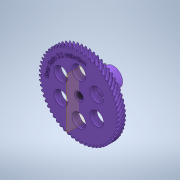
# Autodesk Inventor part: Spur Gear1
Saved by Autodesk Inventor 2020.2 (Build 242310000, 310)
## iProperties
CustomPartVersion: 1
Created: 2019-11-22
Part Number: Spur Gear1
Material: Steel
Document SubType Name: Modeling
Designer: steele
Categories: <?xml version="1.0" encoding="UTF-16"?> <MemberInstance><Categories><FamilyTemplate><FamilyTemplateParameter ValueType="xs:double" Id="1" ObjectReferenceKey="da_z" ObjectType="kUserParameterObject"/><FamilyTemplateParameter ValueType="xs:double" Id="2" ObjectReferenceKey="da_b" ObjectType="kUserParameterObject"/><FamilyTemplateParameter ValueType="xs:double" Id="3" ObjectReferenceKey="da_beta" ObjectType="kUserParameterObject"/><FamilyTemplateParameter ValueType="xs:double" Id="4" ObjectReferenceKey="da_da" ObjectType="kUserParameterObject"/><FamilyTemplateParameter ValueType="xs:double" Id="5" ObjectReferenceKey="da_aw" ObjectType="kUserParameterObject"/><FamilyTemplateParameter ValueType="xs:string" Id="6" ObjectReferenceKey="EAIAABAAAAC/AAAAAAAAAIAAAAAAAAAA" ObjectType="83910656" SubObjectId="SurfaceGeometry"/></FamilyTemplate><ParamToTemplateMap><ParamToTemplate CategoryParameter="//CategoryParameter[@InternalName='046C89C9-8512-4d59-83FE-43B91F4F132A']" TemplateParameter="1"/><ParamToTemplate CategoryParameter="//CategoryParameter[@InternalName='2552DF32-E462-4b46-AEBF-C6C7768E72AC']" TemplateParameter="2"/><ParamToTemplate CategoryParameter="//CategoryParameter[@InternalName='C9EE641D-15FC-4fae-A226-E94C4372FDD7']" TemplateParameter="3"/><ParamToTemplate><ParamToTemplate CategoryParameter="//CategoryParameter[@InternalName='00B6519A-459B-49c7-AD84-2E56D39A5744']" ConstantValue="0.000000"/></ParamToTemplate><ParamToTemplate><ParamToTemplate CategoryParameter="//CategoryParameter[@InternalName='04B31F0E-C7A6-4894-AA32-9629BEFACF47']" ConstantValue="1.000000"/></ParamToTemplate><ParamToTemplate><ParamToTemplate CategoryParameter="//CategoryParameter[@InternalName='43CBEC2E-7847-49e7-A936-2F7889FCB2D9']" ConstantValue="0.250000"/></ParamToTemplate><ParamToTemplate><ParamToTemplate CategoryParameter="//CategoryParameter[@InternalName='B1EFC894-105D-4ebd-86BF-FA20ED196853']" ConstantValue="0.350000"/></ParamToTemplate><ParamToTemplate><ParamToTemplate CategoryParameter="//CategoryParameter[@InternalName='51175063-3D10-4879-93E8-6246FE8B403D']" ConstantValue="2061532430.657340"/></ParamToTemplate><ParamToTemplate><ParamToTemplate CategoryParameter="//CategoryParameter[@InternalName='A3A52E27-4454-46a9-B0BD-C932399B70AF']" ConstantValue="0.300000"/></ParamToTemplate><ParamToTemplate><ParamToTemplate CategoryParameter="//CategoryParameter[@InternalName='91B76062-C214-41d9-B1B9-14D2AB99603D']" ConstantValue="0.127000"/></ParamToTemplate><ParamToTemplate><ParamToTemplate CategoryParameter="//CategoryParameter[@InternalName='374E806E-8B8A-4dda-A9AA-1039D6500AD2']" ConstantValue="7.874016"/></ParamToTemplate><ParamToTemplate><ParamToTemplate CategoryParameter="//CategoryParameter[@InternalName='2D373A89-B862-43d6-8D0B-0CBF12AB9F6C']" ConstantValue="0.349066"/></ParamToTemplate><ParamToTemplate CategoryParameter="//CategoryParameter[@InternalName='37777632-D6A2-4fac-9D53-DB8ACD95C989']" TemplateParameter="4"/><ParamToTemplate CategoryParameter="//CategoryParameter[@InternalName='FD1017F1-B727-4f7e-9707-0F86F1FF9423']" TemplateParameter="5"/><ParamToTemplate><ParamToTemplate CategoryParameter="//CategoryParameter[@InternalName='9E1B4470-B2D3-4ff1-B813-535BB4CDF51A']" ConstantValue="3523220.976809"/></ParamToTemplate><ParamToTemplate><ParamToTemplate CategoryParameter="//CategoryParameter[@InternalName='F8452263-BFF6-458c-9FB1-07C4B99E95CD']" ConstantValue="11397033.805607"/></ParamToTemplate><ParamToTemplate><ParamToTemplate CategoryParameter="//CategoryParameter[@InternalName='3E3BB259-FD49-497f-8171-6EBC954A3479']" ConstantValue="2.000000"/></ParamToTemplate><ParamToTemplate CategoryParameter="//CategoryParameter[@InternalName='27C3BAF2-7550-4e4b-AE2C-0DB134B7D9B7']" TemplateParameter="6"/></ParamToTemplateMap><Category DisplayName="Gear" InternalName="DC85795E-93AB-48d5-8EEE-5A27447B64BD" Mnemonic="Gear"><CategoryParameter DisplayName="z" InternalName="046C89C9-8512-4d59-83FE-43B91F4F132A" Mnemonic="z"/><CategoryParameter DisplayName="b" InternalName="2552DF32-E462-4b46-AEBF-C6C7768E72AC" Mnemonic="b"/><CategoryParameter DisplayName="||b|" InternalName="C9EE641D-15FC-4fae-A226-E94C4372FDD7" Mnemonic="beta"/><CategoryParameter DisplayName="x" InternalName="00B6519A-459B-49c7-AD84-2E56D39A5744" Mnemonic="x"/><CategoryParameter DisplayName="a*" InternalName="04B31F0E-C7A6-4894-AA32-9629BEFACF47" Mnemonic="a"/><CategoryParameter DisplayName="c*" InternalName="43CBEC2E-7847-49e7-A936-2F7889FCB2D9" Mnemonic="c"/><CategoryParameter DisplayName="r|.f|*" InternalName="B1EFC894-105D-4ebd-86BF-FA20ED196853" Mnemonic="rf"/><CategoryParameter DisplayName="E" InternalName="51175063-3D10-4879-93E8-6246FE8B403D" Mnemonic="E"/><CategoryParameter DisplayName="||m|" InternalName="A3A52E27-4454-46a9-B0BD-C932399B70AF" Mnemonic="mi"/><Category DisplayName="SpurGear" InternalName="26C5A22E-A91E-4dfd-A3B3-23CCAFAE1764" Mnemonic="SpurGear"><CategoryParameter DisplayName="m" InternalName="91B76062-C214-41d9-B1B9-14D2AB99603D" Mnemonic="m"/><CategoryParameter DisplayName="P" InternalName="374E806E-8B8A-4dda-A9AA-1039D6500AD2" Mnemonic="PP"/><CategoryParameter DisplayName="||a|" InternalName="2D373A89-B862-43d6-8D0B-0CBF12AB9F6C" Mnemonic="alpha"/><CategoryParameter DisplayName="d|.a|" InternalName="37777632-D6A2-4fac-9D53-DB8ACD95C989" Mnemonic="da"/><CategoryParameter DisplayName="a|.w|" InternalName="FD1017F1-B727-4f7e-9707-0F86F1FF9423" Mnemonic="aw"/><CategoryParameter DisplayName="||s||.Flim|" InternalName="9E1B4470-B2D3-4ff1-B813-535BB4CDF51A" Mnemonic="sFlim"/><CategoryParameter DisplayName="||s||.Hlim|" InternalName="F8452263-BFF6-458c-9FB1-07C4B99E95CD" Mnemonic="sHlim"/><CategoryParameter DisplayName="type" InternalName="3E3BB259-FD49-497f-8171-6EBC954A3479" Mnemonic="type"/><CategoryParameter DisplayName="PitchDiameter" InternalName="27C3BAF2-7550-4e4b-AE2C-0DB134B7D9B7" Mnemonic="IDS_PITCHDIAM"/></Category></Category></Categories></MemberInstance>
Density: 1 g/cm^3
Appearance: Violet
Author: steele
Autodesk Inventor part; units mm, degrees
(part 1 of 2)
ref_plane "XZ Plane" through (0, 0, 0) normal (0, 1, 0) x (-1, 0, 0)
ref_plane "XY Plane" through (0, 0, 0) normal (0, 0, 1) x (1, 0, 0)
sketch "Sketch1" plane through (0, 0, 0) normal (0, 0, 1) x (1, 0, 0)
  circle A0 centre (0, 0) radius 55.1515
  dimension "d0" = 110.3031
  constraints: 1 centre point
  measures "d0" diameter of A0
extrude "Extrusion1" add sketch "Sketch1" along normal blind 9.525
sketch "Sketch2" plane through (0, 0, 0) normal (0, 0, -1) x (-1, 0, 0)
  circle A0 centre (0, 0) radius 55.1515 projected
  circle A1 centre (0, 0) radius 53.8815
  dimension "d3" = 107.7631
  constraints: 1 centre point, 1 coincident
  measures "d3" diameter of A1
surface extrude "Pitch Diameter" sketch "Sketch2" against normal through all shown no curves A1
ref_plane "Work Plane1" through (0, 0, 0) normal (1, 0, 0) x (0, 1, 0)
ref_plane "Work Plane2" through (0, 0, 0) normal (0.9986295, 0.052336, 0) x (0, 0, 1)
ref_plane "Work Plane3" through (0, 0, 4.7625) normal (0, 0, -1) x (-1, 0, 0)
spur gear teeth "Spur Gear" teeth 60 pitch diameter 107.7631 tip diameter 110.3031 root diameter 104.5881 face width 9.525 helix angle 45 hand left start plane through (0, 0, 0) normal (0, 0, -1) x (-1, 0, 0)
sketch "Sketch3" plane through (0, 0, 0) normal (0, 0, -1) x (-1, 0, 0)
  circle A0 centre (0, 0) radius 12.7
  dimension "d20" = 25.4
  constraints: 1 centre point, 1 coincident
  measures "d20" diameter of A0
extrude "Extrusion2" add sketch "Sketch3" along normal blind 38.1
sketch "Sketch4" plane through (0, 0, -38.1) normal (0, 0, -1) x (-1, 0, 0)
  circle A0 centre (0, 0) radius 4.7625
  dimension "d23" = 9.525
  constraints: 1 centre point, 1 coincident
  measures "d23" diameter of A0
extrude "Extrusion3" cut sketch "Sketch4" against normal through all
sketch "Sketch5" plane through (0, 0, 0) normal (0, 0, -1) x (-1, 0, 0)
  circle A0 centre (0, 0) radius 4.7625 projected
  circle A1 centre (0, 28.575) radius 9.525
  circle A2 centre (-24.7467, 14.2875) radius 9.525
  circle A3 centre (-24.7467, -14.2875) radius 9.525
  circle A4 centre (0, -28.575) radius 9.525
  circle A5 centre (24.7467, -14.2875) radius 9.525
  circle A6 centre (24.7467, 14.2875) radius 9.525
  dimension "d27" = 19.05
  dimension "d30" = 360
  constraints: 6 centre point, 2 coincident, 17 other
  measures "d27" diameter of A1
extrude "Extrusion4" cut sketch "Sketch5" against normal through all contours A1 | A2 | A3 | A4 | A5 | A6
fillet "Fillet1" radius 1.5875 2 edges at (4.7625, 0, 9.525) (4.7625, 0, -38.1)
sketch "Sketch6" plane through (0, 0, 9.525) normal (0, 0, 1) x (1, 0, 0)
  circle A0 centre (0, 0) radius 4.7625 construction
  circle A1 centre (0, 0) radius 44.45 construction
  spline S0 degree 2 poles (-41.7293, 2.6333) (-41.7593, 2.0949) (-42.1378, 1.2212) (-42.4885, 0.9192) knots 0 0 0 1 2 2 2
  spline S1 degree 2 poles (-42.4885, 0.9192) (-42.8434, 0.6173) (-43.8571, 0.3315) (-44.5024, 0.3674) knots 0 0 0 1 2 2 2
  spline S2 degree 2 poles (-44.5024, 0.3674) (-45.1149, 0.4015) (-46.0657, 0.8007) (-46.3931, 1.1406) knots 0 0 0 1 2 2 2
  spline S3 degree 2 poles (-46.3931, 1.1406) (-46.7089, 1.4674) (-47.0203, 2.3918) (-46.9903, 2.9302) knots 0 0 0 1 2 2 2
  spline S4 degree 2 poles (-46.9903, 2.9302) (-46.9759, 3.1892) (-46.8759, 3.6536) (-46.7982, 3.8637) knots 0 0 0 1 2 2 2
  spline S5 degree 2 poles (-46.7982, 3.8637) (-46.7393, 4.0336) (-46.5351, 4.4428) (-46.4622, 4.5666) knots 0 0 0 1 2 2 2
  line L0 (-46.4622, 4.5666) -> (-45.6484, 4.5213)
  line L1 (-45.6484, 4.5213) -> (-45.6516, 4.4637)
  spline S6 degree 2 poles (-45.6516, 4.4637) (-45.7697, 4.3425) (-45.9859, 4.0865) (-46.1148, 3.8463) knots 0 0 0 1 2 2 2
  spline S7 degree 2 poles (-46.1148, 3.8463) (-46.229, 3.6465) (-46.3941, 3.1238) (-46.411, 2.8196) knots 0 0 0 1 2 2 2
  spline S8 degree 2 poles (-46.411, 2.8196) (-46.4517, 2.088) (-45.4005, 1.1224) (-44.4839, 1.0714) knots 0 0 0 1 2 2 2
  spline S9 degree 2 poles (-44.4839, 1.0714) (-43.9742, 1.0431) (-43.1964, 1.2389) (-42.9208, 1.4504) knots 0 0 0 1 2 2 2
  spline S10 degree 2 poles (-42.9208, 1.4504) (-42.6456, 1.6536) (-42.3359, 2.2548) (-42.3144, 2.6412) knots 0 0 0 1 2 2 2
  spline S11 degree 2 poles (-42.3144, 2.6412) (-42.2986, 2.9248) (-42.3492, 3.4966) (-42.4207, 3.6943) knots 0 0 0 1 2 2 2
  line L2 (-42.4207, 3.6943) -> (-43.7319, 3.7673)
  line L3 (-43.7319, 3.7673) -> (-43.7973, 2.5917)
  line L4 (-43.7973, 2.5917) -> (-44.3892, 2.6247)
  line L5 (-44.3892, 2.6247) -> (-44.2867, 4.4661)
  line L6 (-44.2867, 4.4661) -> (-42.0713, 4.3428)
  spline S12 degree 2 poles (-42.0713, 4.3428) (-42.0208, 4.2122) (-41.8683, 3.7667) (-41.8252, 3.5787) knots 0 0 0 1 2 2 2
  spline S13 degree 2 poles (-41.8252, 3.5787) (-41.7651, 3.3239) (-41.7136, 2.917) (-41.7293, 2.6333) knots 0 0 0 1 2 2 2
  spline S14 degree 2 poles (-41.2786, 6.7356) (-41.4197, 5.8327) (-42.5875, 4.9985) (-43.523, 5.1447) knots 0 0 0 1 2 2 2
  spline S15 degree 2 poles (-43.523, 5.1447) (-44.4422, 5.2883) (-45.3816, 6.4226) (-45.2602, 7.1995) knots 0 0 0 1 2 2 2
  spline S16 degree 2 poles (-45.2602, 7.1995) (-45.2056, 7.5493) (-44.9177, 8.0584) (-44.671, 8.224) knots 0 0 0 1 2 2 2
  spline S17 degree 2 poles (-44.671, 8.224) (-44.4236, 8.3937) (-43.7676, 8.5121) (-43.3162, 8.4415) knots 0 0 0 1 2 2 2
  line L7 (-43.3162, 8.4415) -> (-42.9704, 8.3875)
  line L8 (-42.9704, 8.3875) -> (-43.3778, 5.7803)
  spline S18 degree 2 poles (-43.3778, 5.7803) (-42.723, 5.678) (-41.9245, 6.2282) (-41.833, 6.8139) knots 0 0 0 1 2 2 2
  spline S19 degree 2 poles (-41.833, 6.8139) (-41.8006, 7.0214) (-41.8312, 7.4386) (-41.879, 7.6128) knots 0 0 0 1 2 2 2
  spline S20 degree 2 poles (-41.879, 7.6128) (-41.9337, 7.7963) (-42.0391, 8.0545) (-42.0922, 8.1419) knots 0 0 0 1 2 2 2
  line L9 (-42.0922, 8.1419) -> (-42.0864, 8.1785)
  line L10 (-42.0864, 8.1785) -> (-41.395, 8.0705)
  spline S21 degree 2 poles (-41.395, 8.0705) (-41.3674, 7.9537) (-41.2894, 7.5998) (-41.2731, 7.4639) knots 0 0 0 1 2 2 2
  spline S22 degree 2 poles (-41.2731, 7.4639) (-41.2488, 7.2726) (-41.243, 6.9634) (-41.2786, 6.7356) knots 0 0 0 1 2 2 2
  spline S23 degree 2 poles (-43.5511, 7.8449) (-43.8086, 7.8768) (-44.1993, 7.8295) (-44.3413, 7.7475) knots 0 0 0 1 2 2 2
  spline S24 degree 2 poles (-44.3413, 7.7475) (-44.5008, 7.66) (-44.7053, 7.3377) (-44.7453, 7.0815) knots 0 0 0 1 2 2 2
  spline S25 degree 2 poles (-44.7453, 7.0815) (-44.7847, 6.8293) (-44.6895, 6.452) (-44.566, 6.2827) knots 0 0 0 1 2 2 2
  spline S26 degree 2 poles (-44.566, 6.2827) (-44.4378, 6.1168) (-44.0986, 5.9138) (-43.8618, 5.856) knots 0 0 0 1 2 2 2
  line L11 (-43.8618, 5.856) -> (-43.5511, 7.8449)
  spline S27 degree 2 poles (-40.8932, 10.8969) (-40.8561, 10.8071) (-40.7195, 10.5019) (-40.6893, 10.3672) knots 0 0 0 1 2 2 2
  spline S28 degree 2 poles (-40.6893, 10.3672) (-40.6419, 10.1816) (-40.6261, 9.8511) (-40.6953, 9.5714) knots 0 0 0 1 2 2 2
  spline S29 degree 2 poles (-40.6953, 9.5714) (-40.7517, 9.3436) (-41.0254, 8.9745) (-41.2198, 8.8573) knots 0 0 0 1 2 2 2
  spline S30 degree 2 poles (-41.2198, 8.8573) (-41.4082, 8.747) (-41.9003, 8.6779) (-42.1481, 8.7392) knots 0 0 0 1 2 2 2
  spline S31 degree 2 poles (-42.1481, 8.7392) (-42.5317, 8.8341) (-42.9951, 9.2923) (-43.0639, 9.6825) knots 0 0 0 1 2 2 2
  spline S32 degree 2 poles (-43.0639, 9.6825) (-43.1307, 10.0298) (-43.0289, 10.9037) (-42.9353, 11.4022) knots 0 0 0 1 2 2 2
  line L12 (-42.9353, 11.4022) -> (-43.0552, 11.4318)
  spline S33 degree 2 poles (-43.0552, 11.4318) (-43.2709, 11.4852) (-43.5713, 11.4196) (-43.6769, 11.3185) knots 0 0 0 1 2 2 2
  spline S34 degree 2 poles (-43.6769, 11.3185) (-43.7825, 11.2174) (-43.9155, 10.8856) (-43.961, 10.7018) knots 0 0 0 1 2 2 2
  spline S35 degree 2 poles (-43.961, 10.7018) (-44.0144, 10.486) (-44.0309, 9.8709) (-43.9792, 9.5485) knots 0 0 0 1 2 2 2
  line L13 (-43.9792, 9.5485) -> (-43.9881, 9.5126)
  line L14 (-43.9881, 9.5126) -> (-44.6235, 9.6698)
  spline S36 degree 2 poles (-44.6235, 9.6698) (-44.6289, 9.8535) (-44.5896, 10.5265) (-44.5115, 10.8422) knots 0 0 0 1 2 2 2
  spline S37 degree 2 poles (-44.5115, 10.8422) (-44.4165, 11.2259) (-44.1671, 11.7197) (-43.9598, 11.8889) knots 0 0 0 1 2 2 2
  spline S38 degree 2 poles (-43.9598, 11.8889) (-43.7576, 12.0552) (-43.2246, 12.1353) (-42.8769, 12.0493) knots 0 0 0 1 2 2 2
  line L15 (-42.8769, 12.0493) -> (-40.3473, 11.4234)
  line L16 (-40.3473, 11.4234) -> (-40.5016, 10.8)
  line L17 (-40.5016, 10.8) -> (-40.8932, 10.8969)
  line L18 (-41.4127, 11.0254) -> (-42.4397, 11.2796)
  spline S39 degree 2 poles (-42.4397, 11.2796) (-42.4751, 11.0508) (-42.5743, 10.3587) (-42.5628, 10.131) knots 0 0 0 1 2 2 2
  spline S40 degree 2 poles (-42.5628, 10.131) (-42.5482, 9.8645) (-42.3126, 9.4627) (-42.0328, 9.3935) knots 0 0 0 1 2 2 2
  spline S41 degree 2 poles (-42.0328, 9.3935) (-41.7131, 9.3144) (-41.3004, 9.5939) (-41.2154, 9.9376) knots 0 0 0 1 2 2 2
  spline S42 degree 2 poles (-41.2154, 9.9376) (-41.1432, 10.2293) (-41.2763, 10.7712) (-41.4127, 11.0254) knots 0 0 0 1 2 2 2
  line L19 (-42.4182, 15.1761) -> (-42.4284, 15.1448)
  spline S43 degree 2 poles (-42.4284, 15.1448) (-42.471, 15.0808) (-42.5288, 14.9308) (-42.5634, 14.8252) knots 0 0 0 1 2 2 2
  spline S44 degree 2 poles (-42.5634, 14.8252) (-42.6441, 14.5787) (-42.5877, 14.0231) (-42.4482, 13.7349) knots 0 0 0 1 2 2 2
  line L20 (-42.4482, 13.7349) -> (-39.8777, 12.8934)
  line L21 (-39.8777, 12.8934) -> (-40.0775, 12.2831)
  line L22 (-40.0775, 12.2831) -> (-43.7004, 13.469)
  line L23 (-43.7004, 13.469) -> (-43.5006, 14.0794)
  line L24 (-43.5006, 14.0794) -> (-42.9607, 13.9026)
  spline S45 degree 2 poles (-42.9607, 13.9026) (-43.1492, 14.3325) (-43.2291, 14.9088) (-43.1522, 15.1435) knots 0 0 0 1 2 2 2
  spline S46 degree 2 poles (-43.1522, 15.1435) (-43.1215, 15.2374) (-43.0829, 15.3288) (-43.052, 15.3836) knots 0 0 0 1 2 2 2
  line L25 (-43.052, 15.3836) -> (-42.4182, 15.1761)
  line L26 (-36.7442, 20.2855) -> (-37.1257, 19.496)
  line L27 (-37.1257, 19.496) -> (-39.6442, 18.9298)
  line L28 (-39.6442, 18.9298) -> (-39.9809, 18.2329)
  line L29 (-39.9809, 18.2329) -> (-38.161, 17.3535)
  line L30 (-38.161, 17.3535) -> (-38.4547, 16.7456)
  line L31 (-38.4547, 16.7456) -> (-43.0287, 18.9558)
  line L32 (-43.0287, 18.9558) -> (-42.4592, 20.1345)
  spline S47 degree 2 poles (-42.4592, 20.1345) (-42.2693, 20.5274) (-41.9279, 21.0163) (-41.6558, 21.182) knots 0 0 0 1 2 2 2
  spline S48 degree 2 poles (-41.6558, 21.182) (-41.3837, 21.3477) (-40.7638, 21.391) (-40.4043, 21.2173) knots 0 0 0 1 2 2 2
  spline S49 degree 2 poles (-40.4043, 21.2173) (-39.9039, 20.9755) (-39.4727, 20.1362) (-39.521, 19.62) knots 0 0 0 1 2 2 2
  line L33 (-39.521, 19.62) -> (-36.7442, 20.2855)
  spline S50 degree 2 poles (-40.6624, 20.5602) (-40.8625, 20.6569) (-41.2382, 20.6647) (-41.41, 20.5648) knots 0 0 0 1 2 2 2
  spline S51 degree 2 poles (-41.41, 20.5648) (-41.5579, 20.4763) (-41.7949, 20.1656) (-41.9167, 19.9135) knots 0 0 0 1 2 2 2
  line L34 (-41.9167, 19.9135) -> (-42.2086, 19.3093)
  line L35 (-42.2086, 19.3093) -> (-40.4888, 18.4783)
  line L36 (-40.4888, 18.4783) -> (-40.2308, 19.012)
  spline S52 degree 2 poles (-40.2308, 19.012) (-40.1037, 19.2752) (-39.994, 19.7388) (-40.0687, 19.9533) knots 0 0 0 1 2 2 2
  spline S53 degree 2 poles (-40.0687, 19.9533) (-40.1302, 20.1476) (-40.4252, 20.4456) (-40.6624, 20.5602) knots 0 0 0 1 2 2 2
  spline S54 degree 2 poles (-35.78, 22.6006) (-35.7713, 22.5039) (-35.7321, 22.1718) (-35.7434, 22.0342) knots 0 0 0 1 2 2 2
  spline S55 degree 2 poles (-35.7434, 22.0342) (-35.7535, 21.8429) (-35.837, 21.5228) (-35.9866, 21.2765) knots 0 0 0 1 2 2 2
  spline S56 degree 2 poles (-35.9866, 21.2765) (-36.1083, 21.0759) (-36.4796, 20.8053) (-36.7002, 20.7513) knots 0 0 0 1 2 2 2
  spline S57 degree 2 poles (-36.7002, 20.7513) (-36.913, 20.7023) (-37.4032, 20.7832) (-37.6214, 20.9156) knots 0 0 0 1 2 2 2
  spline S58 degree 2 poles (-37.6214, 20.9156) (-37.9593, 21.1206) (-38.2649, 21.6962) (-38.2141, 22.0892) knots 0 0 0 1 2 2 2
  spline S59 degree 2 poles (-38.2141, 22.0892) (-38.1742, 22.4406) (-37.8164, 23.2443) (-37.5783, 23.6921) knots 0 0 0 1 2 2 2
  line L37 (-37.5783, 23.6921) -> (-37.6839, 23.7562)
  spline S60 degree 2 poles (-37.6839, 23.7562) (-37.8739, 23.8716) (-38.1802, 23.8985) (-38.3111, 23.8335) knots 0 0 0 1 2 2 2
  spline S61 degree 2 poles (-38.3111, 23.8335) (-38.4421, 23.7686) (-38.668, 23.4915) (-38.7663, 23.3297) knots 0 0 0 1 2 2 2
  spline S62 degree 2 poles (-38.7663, 23.3297) (-38.8816, 23.1396) (-39.0809, 22.5575) (-39.1277, 22.2343) knots 0 0 0 1 2 2 2
  line L38 (-39.1277, 22.2343) -> (-39.1469, 22.2027)
  line L39 (-39.1469, 22.2027) -> (-39.7065, 22.5423)
  spline S63 degree 2 poles (-39.7065, 22.5423) (-39.6568, 22.7193) (-39.4185, 23.3499) (-39.2498, 23.6279) knots 0 0 0 1 2 2 2
  spline S64 degree 2 poles (-39.2498, 23.6279) (-39.0447, 23.9658) (-38.6593, 24.3627) (-38.411, 24.4624) knots 0 0 0 1 2 2 2
  spline S65 degree 2 poles (-38.411, 24.4624) (-38.1683, 24.5607) (-37.6357, 24.4782) (-37.3296, 24.2924) knots 0 0 0 1 2 2 2
  line L40 (-37.3296, 24.2924) -> (-35.1019, 22.9403)
  line L41 (-35.1019, 22.9403) -> (-35.4351, 22.3913)
  line L42 (-35.4351, 22.3913) -> (-35.78, 22.6006)
  line L43 (-36.2375, 22.8783) -> (-37.1419, 23.4273)
  spline S66 degree 2 poles (-37.1419, 23.4273) (-37.2439, 23.2195) (-37.5451, 22.5885) (-37.602, 22.3678) knots 0 0 0 1 2 2 2
  spline S67 degree 2 poles (-37.602, 22.3678) (-37.6676, 22.109) (-37.5626, 21.6552) (-37.3162, 21.5057) knots 0 0 0 1 2 2 2
  spline S68 degree 2 poles (-37.3162, 21.5057) (-37.0347, 21.3348) (-36.5574, 21.4785) (-36.3737, 21.7812) knots 0 0 0 1 2 2 2
  spline S69 degree 2 poles (-36.3737, 21.7812) (-36.2178, 22.0381) (-36.1832, 22.5949) (-36.2375, 22.8783) knots 0 0 0 1 2 2 2
  spline S70 degree 2 poles (-33.859, 24.5766) (-34.1616, 24.1503) (-34.9891, 24.0156) (-35.5161, 24.3896) knots 0 0 0 1 2 2 2
  line L44 (-35.5161, 24.3896) -> (-37.2384, 25.6118)
  line L45 (-37.2384, 25.6118) -> (-37.4886, 25.2593)
  line L46 (-37.4886, 25.2593) -> (-37.9217, 25.5666)
  line L47 (-37.9217, 25.5666) -> (-37.6715, 25.9191)
  line L48 (-37.6715, 25.9191) -> (-38.5646, 26.5528)
  line L49 (-38.5646, 26.5528) -> (-38.1929, 27.0766)
  line L50 (-38.1929, 27.0766) -> (-37.2999, 26.4429)
  line L51 (-37.2999, 26.4429) -> (-36.6162, 27.4064)
  line L52 (-36.6162, 27.4064) -> (-36.1831, 27.0991)
  line L53 (-36.1831, 27.0991) -> (-36.8668, 26.1355)
  line L54 (-36.8668, 26.1355) -> (-35.3862, 25.0849)
  spline S71 degree 2 poles (-35.3862, 25.0849) (-35.1512, 24.9182) (-34.8808, 24.7515) (-34.7295, 24.73) knots 0 0 0 1 2 2 2
  spline S72 degree 2 poles (-34.7295, 24.73) (-34.5988, 24.7079) (-34.3513, 24.8503) (-34.2227, 25.0316) knots 0 0 0 1 2 2 2
  spline S73 degree 2 poles (-34.2227, 25.0316) (-34.1322, 25.1592) (-34.0402, 25.4523) (-34.0256, 25.5227) knots 0 0 0 1 2 2 2
  line L55 (-34.0256, 25.5227) -> (-34.0042, 25.5529)
  line L56 (-34.0042, 25.5529) -> (-33.5341, 25.2194)
  spline S74 degree 2 poles (-33.5341, 25.2194) (-33.5987, 25.0431) (-33.7661, 24.7076) (-33.859, 24.5766) knots 0 0 0 1 2 2 2
  line L57 (-32.8054, 26.0836) -> (-33.2013, 25.5779)
  line L58 (-33.2013, 25.5779) -> (-36.2032, 27.9274)
  line L59 (-36.2032, 27.9274) -> (-35.8074, 28.4331)
  line L60 (-35.8074, 28.4331) -> (-32.8054, 26.0836)
  line L61 (-36.2787, 28.8595) -> (-36.7278, 28.2857)
  line L62 (-36.7278, 28.2857) -> (-37.253, 28.6968)
  line L63 (-37.253, 28.6968) -> (-36.8039, 29.2706)
  line L64 (-36.8039, 29.2706) -> (-36.2787, 28.8595)
  spline S75 degree 2 poles (-31.5659, 30.4357) (-30.847, 29.7945) (-30.6802, 28.4045) (-31.1953, 27.8269) knots 0 0 0 1 2 2 2
  spline S76 degree 2 poles (-31.1953, 27.8269) (-31.7242, 27.234) (-33.1378, 27.2757) (-33.8321, 27.895) knots 0 0 0 1 2 2 2
  spline S77 degree 2 poles (-33.8321, 27.895) (-34.5448, 28.5307) (-34.7096, 29.9354) (-34.2, 30.5069) knots 0 0 0 1 2 2 2
  spline S78 degree 2 poles (-34.2, 30.5069) (-33.6848, 31.0844) (-32.2818, 31.0742) (-31.5659, 30.4357) knots 0 0 0 1 2 2 2
  spline S79 degree 2 poles (-32.0071, 29.9411) (-32.5601, 30.4343) (-33.4567, 30.5114) (-33.7883, 30.1397) knots 0 0 0 1 2 2 2
  spline S80 degree 2 poles (-33.7883, 30.1397) (-34.1198, 29.7679) (-33.9439, 28.8829) (-33.3909, 28.3896) knots 0 0 0 1 2 2 2
  spline S81 degree 2 poles (-33.3909, 28.3896) (-32.8533, 27.9101) (-31.9386, 27.8224) (-31.607, 28.1941) knots 0 0 0 1 2 2 2
  spline S82 degree 2 poles (-31.607, 28.1941) (-31.2782, 28.5628) (-31.4603, 29.4533) (-32.0071, 29.9411) knots 0 0 0 1 2 2 2
  spline S83 degree 2 poles (-30.0788, 35.4728) (-30.2205, 35.3535) (-30.4425, 35.0482) (-30.5328, 34.8807) knots 0 0 0 1 2 2 2
  spline S84 degree 2 poles (-30.5328, 34.8807) (-30.6137, 34.7211) (-30.7041, 34.4513) (-30.7341, 34.3399) knots 0 0 0 1 2 2 2
  line L65 (-30.7341, 34.3399) -> (-30.7656, 34.3134)
  line L66 (-30.7656, 34.3134) -> (-31.2296, 34.8646)
  spline S85 degree 2 poles (-31.2296, 34.8646) (-31.1364, 35.0991) (-30.6784, 35.7376) (-30.417, 35.9576) knots 0 0 0 1 2 2 2
  spline S86 degree 2 poles (-30.417, 35.9576) (-30.1525, 36.1803) (-29.6687, 36.4047) (-29.4126, 36.4265) knots 0 0 0 1 2 2 2
  spline S87 degree 2 poles (-29.4126, 36.4265) (-29.1391, 36.4468) (-28.6632, 36.2394) (-28.4617, 36.0001) knots 0 0 0 1 2 2 2
  spline S88 degree 2 poles (-28.4617, 36.0001) (-28.1913, 35.6789) (-28.205, 34.8386) (-28.448, 34.5264) knots 0 0 0 1 2 2 2
  line L67 (-28.448, 34.5264) -> (-28.4161, 34.4886)
  spline S89 degree 2 poles (-28.4161, 34.4886) (-28.2721, 34.5668) (-27.8964, 34.6894) (-27.6813, 34.6768) knots 0 0 0 1 2 2 2
  spline S90 degree 2 poles (-27.6813, 34.6768) (-27.4688, 34.6673) (-27.0207, 34.4419) (-26.8059, 34.1868) knots 0 0 0 1 2 2 2
  spline S91 degree 2 poles (-26.8059, 34.1868) (-26.5859, 33.9254) (-26.3916, 33.3302) (-26.4122, 33.0223) knots 0 0 0 1 2 2 2
  spline S92 degree 2 poles (-26.4122, 33.0223) (-26.4337, 32.7028) (-26.7618, 32.1145) (-27.0673, 31.8573) knots 0 0 0 1 2 2 2
  spline S93 degree 2 poles (-27.0673, 31.8573) (-27.3602, 31.6107) (-28.0526, 31.2699) (-28.3301, 31.2031) knots 0 0 0 1 2 2 2
  line L68 (-28.3301, 31.2031) -> (-28.7941, 31.7543)
  line L69 (-28.7941, 31.7543) -> (-28.7563, 31.7861)
  spline S94 degree 2 poles (-28.7563, 31.7861) (-28.4918, 31.8043) (-27.7519, 32.0504) (-27.4779, 32.2811) knots 0 0 0 1 2 2 2
  spline S95 degree 2 poles (-27.4779, 32.2811) (-27.3173, 32.4163) (-27.0809, 32.7875) (-27.0719, 32.9942) knots 0 0 0 1 2 2 2
  spline S96 degree 2 poles (-27.0719, 32.9942) (-27.0661, 33.1982) (-27.1892, 33.5681) (-27.3668, 33.7791) knots 0 0 0 1 2 2 2
  spline S97 degree 2 poles (-27.3668, 33.7791) (-27.5445, 33.9901) (-27.8979, 34.1607) (-28.0745, 34.1467) knots 0 0 0 1 2 2 2
  spline S98 degree 2 poles (-28.0745, 34.1467) (-28.251, 34.1326) (-28.6005, 33.9406) (-28.7769, 33.7921) knots 0 0 0 1 2 2 2
  line L70 (-28.7769, 33.7921) -> (-28.9973, 33.6065)
  line L71 (-28.9973, 33.6065) -> (-29.3605, 34.038)
  line L72 (-29.3605, 34.038) -> (-29.1873, 34.1838)
  spline S99 degree 2 poles (-29.1873, 34.1838) (-28.8378, 34.4781) (-28.6779, 35.1831) (-28.9457, 35.5011) knots 0 0 0 1 2 2 2
  spline S100 degree 2 poles (-28.9457, 35.5011) (-29.0703, 35.6492) (-29.3613, 35.7647) (-29.5057, 35.7508) knots 0 0 0 1 2 2 2
  spline S101 degree 2 poles (-29.5057, 35.7508) (-29.659, 35.7348) (-29.9434, 35.5868) (-30.0788, 35.4728) knots 0 0 0 1 2 2 2
  line L73 (-25.8474, 36.5334) -> (-26.5085, 36.0566)
  line L74 (-26.5085, 36.0566) -> (-27.0768, 36.8445)
  line L75 (-27.0768, 36.8445) -> (-26.4157, 37.3214)
  line L76 (-26.4157, 37.3214) -> (-25.8474, 36.5334)
  line L77 (-24.1857, 34.2296) -> (-24.8468, 33.7528)
  line L78 (-24.8468, 33.7528) -> (-25.4152, 34.5407)
  line L79 (-25.4152, 34.5407) -> (-24.7541, 35.0175)
  line L80 (-24.7541, 35.0175) -> (-24.1857, 34.2296)
  line L81 (-20.7596, 36.432) -> (-22.8724, 35.1368)
  line L82 (-22.8724, 35.1368) -> (-23.1435, 35.579)
  line L83 (-23.1435, 35.579) -> (-22.3573, 36.0609)
  line L84 (-22.3573, 36.0609) -> (-24.1367, 38.9635)
  line L85 (-24.1367, 38.9635) -> (-24.9228, 38.4815)
  line L86 (-24.9228, 38.4815) -> (-25.166, 38.8781)
  spline S102 degree 2 poles (-25.166, 38.8781) (-24.7202, 39.1514) (-24.454, 39.6622) (-24.641, 40.0304) knots 0 0 0 1 2 2 2
  line L87 (-24.641, 40.0304) -> (-24.1918, 40.3058)
  line L88 (-24.1918, 40.3058) -> (-21.7993, 36.403)
  line L89 (-21.7993, 36.403) -> (-21.0307, 36.8742)
  line L90 (-21.0307, 36.8742) -> (-20.7596, 36.432)
  line L91 (-17.3429, 41.5794) -> (-17.3729, 41.5659)
  spline S103 degree 2 poles (-17.3729, 41.5659) (-17.4489, 41.5542) (-17.5987, 41.4959) (-17.7001, 41.4504) knots 0 0 0 1 2 2 2
  spline S104 degree 2 poles (-17.7001, 41.4504) (-17.9367, 41.3441) (-18.3095, 40.9283) (-18.4286, 40.631) knots 0 0 0 1 2 2 2
  line L92 (-18.4286, 40.631) -> (-17.3198, 38.164)
  line L93 (-17.3198, 38.164) -> (-17.9056, 37.9008)
  line L94 (-17.9056, 37.9008) -> (-19.4683, 41.3778)
  line L95 (-19.4683, 41.3778) -> (-18.8826, 41.6411)
  line L96 (-18.8826, 41.6411) -> (-18.6497, 41.1229)
  spline S105 degree 2 poles (-18.6497, 41.1229) (-18.4588, 41.5517) (-18.0866, 41.9988) (-17.8613, 42.1001) knots 0 0 0 1 2 2 2
  spline S106 degree 2 poles (-17.8613, 42.1001) (-17.7711, 42.1406) (-17.6776, 42.1736) (-17.6163, 42.1876) knots 0 0 0 1 2 2 2
  line L97 (-17.6163, 42.1876) -> (-17.3429, 41.5794)
  spline S107 degree 2 poles (-14.0179, 39.4054) (-14.8769, 39.0933) (-16.171, 39.7137) (-16.4944, 40.6036) knots 0 0 0 1 2 2 2
  spline S108 degree 2 poles (-16.4944, 40.6036) (-16.8121, 41.4781) (-16.2719, 42.8482) (-15.5329, 43.1167) knots 0 0 0 1 2 2 2
  spline S109 degree 2 poles (-15.5329, 43.1167) (-15.2001, 43.2376) (-14.6152, 43.2311) (-14.3511, 43.095) knots 0 0 0 1 2 2 2
  spline S110 degree 2 poles (-14.3511, 43.095) (-14.0831, 42.9602) (-13.663, 42.4427) (-13.5069, 42.0132) knots 0 0 0 1 2 2 2
  line L98 (-13.5069, 42.0132) -> (-13.3874, 41.6844)
  line L99 (-13.3874, 41.6844) -> (-15.8676, 40.7832)
  spline S111 degree 2 poles (-15.8676, 40.7832) (-15.6412, 40.1602) (-14.774, 39.7264) (-14.2169, 39.9288) knots 0 0 0 1 2 2 2
  spline S112 degree 2 poles (-14.2169, 39.9288) (-14.0195, 40.0005) (-13.6688, 40.2287) (-13.5394, 40.3546) knots 0 0 0 1 2 2 2
  spline S113 degree 2 poles (-13.5394, 40.3546) (-13.405, 40.491) (-13.2298, 40.708) (-13.1787, 40.7966) knots 0 0 0 1 2 2 2
  line L100 (-13.1787, 40.7966) -> (-13.1439, 40.8092)
  line L101 (-13.1439, 40.8092) -> (-12.9049, 40.1515)
  spline S114 degree 2 poles (-12.9049, 40.1515) (-12.9939, 40.0709) (-13.2662, 39.8319) (-13.3774, 39.752) knots 0 0 0 1 2 2 2
  spline S115 degree 2 poles (-13.3774, 39.752) (-13.5332, 39.6385) (-13.8013, 39.4841) (-14.0179, 39.4054) knots 0 0 0 1 2 2 2
  spline S116 degree 2 poles (-14.1428, 41.9311) (-14.2392, 42.172) (-14.4691, 42.4915) (-14.6094, 42.5763) knots 0 0 0 1 2 2 2
  spline S117 degree 2 poles (-14.6094, 42.5763) (-14.7631, 42.6737) (-15.144, 42.6974) (-15.3877, 42.6088) knots 0 0 0 1 2 2 2
  spline S118 degree 2 poles (-15.3877, 42.6088) (-15.6276, 42.5216) (-15.9122, 42.2562) (-16.0009, 42.0663) knots 0 0 0 1 2 2 2
  spline S119 degree 2 poles (-16.0009, 42.0663) (-16.0843, 41.8739) (-16.0985, 41.4789) (-16.0349, 41.2436) knots 0 0 0 1 2 2 2
  line L102 (-16.0349, 41.2436) -> (-14.1428, 41.9311)
  line L103 (-9.3028, 40.8907) -> (-9.9237, 40.7265)
  line L104 (-9.9237, 40.7265) -> (-10.0227, 41.1006)
  spline S120 degree 2 poles (-10.0227, 41.1006) (-10.1343, 40.9433) (-10.3032, 40.7283) (-10.4285, 40.6227) knots 0 0 0 1 2 2 2
  spline S121 degree 2 poles (-10.4285, 40.6227) (-10.543, 40.5243) (-10.8077, 40.3819) (-10.9947, 40.3324) knots 0 0 0 1 2 2 2
  spline S122 degree 2 poles (-10.9947, 40.3324) (-11.2972, 40.2524) (-11.8729, 40.3683) (-12.1162, 40.5637) knots 0 0 0 1 2 2 2
  spline S123 degree 2 poles (-12.1162, 40.5637) (-12.3596, 40.7591) (-12.7481, 41.4228) (-12.8713, 41.8884) knots 0 0 0 1 2 2 2
  spline S124 degree 2 poles (-12.8713, 41.8884) (-12.9997, 42.3739) (-12.9364, 43.1487) (-12.7881, 43.4732) knots 0 0 0 1 2 2 2
  spline S125 degree 2 poles (-12.7881, 43.4732) (-12.6483, 43.7657) (-12.1519, 44.1909) (-11.8375, 44.2741) knots 0 0 0 1 2 2 2
  spline S126 degree 2 poles (-11.8375, 44.2741) (-11.5629, 44.3467) (-11.1203, 44.3318) (-10.8598, 44.2645) knots 0 0 0 1 2 2 2
  line L105 (-10.8598, 44.2645) -> (-11.2809, 45.8564)
  line L106 (-11.2809, 45.8564) -> (-10.6601, 46.0206)
  line L107 (-10.6601, 46.0206) -> (-9.3028, 40.8907)
  line L108 (-10.1606, 41.6219) -> (-10.7239, 43.7511)
  spline S127 degree 2 poles (-10.7239, 43.7511) (-10.9842, 43.8015) (-11.3725, 43.7882) (-11.5834, 43.7324) knots 0 0 0 1 2 2 2
  spline S128 degree 2 poles (-11.5834, 43.7324) (-12.061, 43.606) (-12.4127, 42.7464) (-12.2337, 42.0699) knots 0 0 0 1 2 2 2
  spline S129 degree 2 poles (-12.2337, 42.0699) (-12.061, 41.4172) (-11.465, 40.8382) (-11.0073, 40.9593) knots 0 0 0 1 2 2 2
  spline S130 degree 2 poles (-11.0073, 40.9593) (-10.7645, 41.0235) (-10.33, 41.377) (-10.1606, 41.6219) knots 0 0 0 1 2 2 2
  line L109 (-5.4713, 41.5777) -> (-6.1047, 41.4715)
  line L110 (-6.1047, 41.4715) -> (-6.1741, 41.8856)
  spline S131 degree 2 poles (-6.1741, 41.8856) (-6.4236, 41.5808) (-6.903, 41.2291) (-7.2278, 41.1746) knots 0 0 0 1 2 2 2
  spline S132 degree 2 poles (-7.2278, 41.1746) (-7.4714, 41.1337) (-7.9331, 41.2233) (-8.1207, 41.3713) knots 0 0 0 1 2 2 2
  spline S133 degree 2 poles (-8.1207, 41.3713) (-8.3124, 41.5186) (-8.5802, 42.0205) (-8.6443, 42.4022) knots 0 0 0 1 2 2 2
  line L111 (-8.6443, 42.4022) -> (-9.0535, 44.8422)
  line L112 (-9.0535, 44.8422) -> (-8.4202, 44.9484)
  line L113 (-8.4202, 44.9484) -> (-8.0606, 42.8048)
  spline S134 degree 2 poles (-8.0606, 42.8048) (-8.0102, 42.5043) (-7.8995, 42.118) (-7.7978, 41.9848) knots 0 0 0 1 2 2 2
  spline S135 degree 2 poles (-7.7978, 41.9848) (-7.6962, 41.8516) (-7.4098, 41.7618) (-7.1622, 41.8034) knots 0 0 0 1 2 2 2
  spline S136 degree 2 poles (-7.1622, 41.8034) (-6.9307, 41.8422) (-6.4513, 42.194) (-6.264, 42.4215) knots 0 0 0 1 2 2 2
  line L114 (-6.264, 42.4215) -> (-6.7353, 45.231)
  line L115 (-6.7353, 45.231) -> (-6.1019, 45.3373)
  line L116 (-6.1019, 45.3373) -> (-5.4713, 41.5777)
  spline S137 degree 2 poles (-3.0302, 41.7153) (-3.4241, 41.6832) (-4.0963, 41.8721) (-4.3502, 42.0992) knots 0 0 0 1 2 2 2
  spline S138 degree 2 poles (-4.3502, 42.0992) (-4.6038, 42.3222) (-4.9232, 43.0479) (-4.964, 43.5485) knots 0 0 0 1 2 2 2
  spline S139 degree 2 poles (-4.964, 43.5485) (-5.0048, 44.0491) (-4.7976, 44.8011) (-4.592, 45.0657) knots 0 0 0 1 2 2 2
  spline S140 degree 2 poles (-4.592, 45.0657) (-4.3867, 45.3344) (-3.7396, 45.6556) (-3.354, 45.687) knots 0 0 0 1 2 2 2
  spline S141 degree 2 poles (-3.354, 45.687) (-3.0421, 45.7125) (-2.4451, 45.5835) (-2.2101, 45.487) knots 0 0 0 1 2 2 2
  line L117 (-2.2101, 45.487) -> (-2.1515, 44.769)
  line L118 (-2.1515, 44.769) -> (-2.1885, 44.766)
  spline S142 degree 2 poles (-2.1885, 44.766) (-2.2629, 44.8177) (-2.4883, 44.9481) (-2.6465, 45.0136) knots 0 0 0 1 2 2 2
  spline S143 degree 2 poles (-2.6465, 45.0136) (-2.7872, 45.0683) (-3.1567, 45.1414) (-3.3208, 45.128) knots 0 0 0 1 2 2 2
  spline S144 degree 2 poles (-3.3208, 45.128) (-3.8173, 45.0876) (-4.3592, 44.2875) (-4.3034, 43.6023) knots 0 0 0 1 2 2 2
  spline S145 degree 2 poles (-4.3034, 43.6023) (-4.2489, 42.9335) (-3.605, 42.2301) (-3.088, 42.2723) knots 0 0 0 1 2 2 2
  spline S146 degree 2 poles (-3.088, 42.2723) (-2.7762, 42.2977) (-2.231, 42.6023) (-2.03, 42.8211) knots 0 0 0 1 2 2 2
  line L119 (-2.03, 42.8211) -> (-1.993, 42.8241)
  line L120 (-1.993, 42.8241) -> (-1.9345, 42.1061)
  spline S147 degree 2 poles (-1.9345, 42.1061) (-2.0252, 42.0533) (-2.3021, 41.9026) (-2.4146, 41.8646) knots 0 0 0 1 2 2 2
  spline S148 degree 2 poles (-2.4146, 41.8646) (-2.5747, 41.8019) (-2.8292, 41.7316) (-3.0302, 41.7153) knots 0 0 0 1 2 2 2
  spline S149 degree 2 poles (-0.1787, 41.8379) (-0.7015, 41.8301) (-1.2991, 42.4181) (-1.3087, 43.0644) knots 0 0 0 1 2 2 2
  line L121 (-1.3087, 43.0644) -> (-1.3404, 45.176)
  line L122 (-1.3404, 45.176) -> (-1.7726, 45.1695)
  line L123 (-1.7726, 45.1695) -> (-1.7806, 45.7005)
  line L124 (-1.7806, 45.7005) -> (-1.3484, 45.707)
  line L125 (-1.3484, 45.707) -> (-1.3648, 46.8019)
  line L126 (-1.3648, 46.8019) -> (-0.7227, 46.8115)
  line L127 (-0.7227, 46.8115) -> (-0.7062, 45.7166)
  line L128 (-0.7062, 45.7166) -> (0.4751, 45.7343)
  line L129 (0.4751, 45.7343) -> (0.4831, 45.2033)
  line L130 (0.4831, 45.2033) -> (-0.6983, 45.1856)
  line L131 (-0.6983, 45.1856) -> (-0.6711, 43.3704)
  spline S150 degree 2 poles (-0.6711, 43.3704) (-0.6667, 43.0822) (-0.6414, 42.7656) (-0.5694, 42.6308) knots 0 0 0 1 2 2 2
  spline S151 degree 2 poles (-0.5694, 42.6308) (-0.51, 42.5123) (-0.2489, 42.3968) (-0.0266, 42.4001) knots 0 0 0 1 2 2 2
  spline S152 degree 2 poles (-0.0266, 42.4001) (0.1298, 42.4025) (0.4207, 42.5015) (0.4861, 42.5313) knots 0 0 0 1 2 2 2
  line L132 (0.4861, 42.5313) -> (0.5231, 42.5319)
  line L133 (0.5231, 42.5319) -> (0.5318, 41.9556)
  spline S153 degree 2 poles (0.5318, 41.9556) (0.3514, 41.9035) (-0.0182, 41.8403) (-0.1787, 41.8379) knots 0 0 0 1 2 2 2
  line L134 (1.6596, 41.8784) -> (1.0177, 41.8989)
  line L135 (1.0177, 41.8989) -> (1.1395, 45.709)
  line L136 (1.1395, 45.709) -> (1.7813, 45.6885)
  line L137 (1.7813, 45.6885) -> (1.6596, 41.8784)
  line L138 (1.8468, 46.3207) -> (1.1186, 46.3439)
  line L139 (1.1186, 46.3439) -> (1.1399, 47.0105)
  line L140 (1.1399, 47.0105) -> (1.8681, 46.9872)
  line L141 (1.8681, 46.9872) -> (1.8468, 46.3207)
  spline S154 degree 2 poles (5.9031, 43.4499) (5.8106, 42.4911) (4.7878, 41.5351) (4.0174, 41.6095) knots 0 0 0 1 2 2 2
  spline S155 degree 2 poles (4.0174, 41.6095) (3.2266, 41.6858) (2.425, 42.8509) (2.5143, 43.7769) knots 0 0 0 1 2 2 2
  spline S156 degree 2 poles (2.5143, 43.7769) (2.6061, 44.7276) (3.642, 45.6905) (4.4041, 45.617) knots 0 0 0 1 2 2 2
  spline S157 degree 2 poles (4.4041, 45.617) (5.1745, 45.5426) (5.9952, 44.4047) (5.9031, 43.4499) knots 0 0 0 1 2 2 2
  spline S158 degree 2 poles (5.2434, 43.5136) (5.3145, 44.2512) (4.847, 45.0201) (4.3511, 45.0679) knots 0 0 0 1 2 2 2
  spline S159 degree 2 poles (4.3511, 45.0679) (3.8553, 45.1157) (3.2452, 44.4509) (3.1741, 43.7133) knots 0 0 0 1 2 2 2
  spline S160 degree 2 poles (3.1741, 43.7133) (3.1049, 42.9962) (3.5746, 42.2064) (4.0704, 42.1586) knots 0 0 0 1 2 2 2
  spline S161 degree 2 poles (4.0704, 42.1586) (4.5621, 42.1111) (5.173, 42.7842) (5.2434, 43.5136) knots 0 0 0 1 2 2 2
  line L142 (9.3101, 40.8907) -> (8.6792, 41.0107)
  line L143 (8.6792, 41.0107) -> (9.0851, 43.146)
  spline S162 degree 2 poles (9.0851, 43.146) (9.1343, 43.4049) (9.1703, 43.859) (9.1229, 44.0063) knots 0 0 0 1 2 2 2
  spline S163 degree 2 poles (9.1229, 44.0063) (9.073, 44.1624) (8.8241, 44.3522) (8.5895, 44.3968) knots 0 0 0 1 2 2 2
  spline S164 degree 2 poles (8.5895, 44.3968) (8.355, 44.4414) (7.8098, 44.2852) (7.5328, 44.1283) knots 0 0 0 1 2 2 2
  line L144 (7.5328, 44.1283) -> (7.0008, 41.3297)
  line L145 (7.0008, 41.3297) -> (6.3699, 41.4496)
  line L146 (6.3699, 41.4496) -> (7.0818, 45.1946)
  line L147 (7.0818, 45.1946) -> (7.7127, 45.0747)
  line L148 (7.7127, 45.0747) -> (7.6335, 44.6581)
  spline S165 degree 2 poles (7.6335, 44.6581) (7.965, 44.8591) (8.5617, 45.0222) (8.8691, 44.9638) knots 0 0 0 1 2 2 2
  spline S166 degree 2 poles (8.8691, 44.9638) (9.4191, 44.8593) (9.9036, 44.0129) (9.7721, 43.3213) knots 0 0 0 1 2 2 2
  line L149 (9.7721, 43.3213) -> (9.3101, 40.8907)
  dimension "d35" = 88.9
  constraints: 1 centre point, 1 coincident, 1 other
  measures "d35" diameter of A1
extrude "Extrusion5" cut sketch "Sketch6" against normal blind 3.175